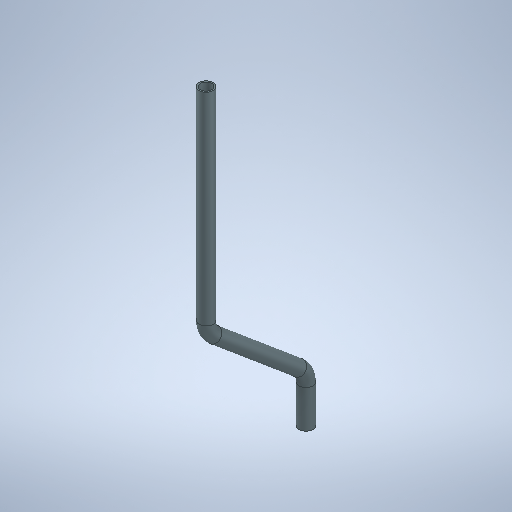
# Autodesk Inventor part: 158 diameter 76
Saved by Autodesk Inventor 2025.1 (Build 291241000, 241)
## iProperties
Created: 2024-08-03
Part Number: 158 diameter 76
Material: Iron, Gray
Document SubType Name: Modeling
Designer: ffogue
Density: 7.15 g/cm^3
Appearance: Lead
Author: ffogue
Autodesk Inventor part; units mm, degrees
ref_plane "YZ Plane" through (0, 0, 0) normal (1, 0, 0) x (0, 1, 0)
ref_plane "XZ Plane" through (0, 0, 0) normal (0, 1, 0) x (-1, 0, 0)
ref_plane "XY Plane" through (0, 0, 0) normal (0, 0, 1) x (1, 0, 0)
sketch "Sketch1" plane through (0, 0, 0) normal (0, 0, 1) x (1, 0, 0)
  circle A0 centre (0, 0) radius 2.5
  dimension "d0" = 5
  constraints: 1 centre point, 1 coincident
  measures "d0" diameter of A0
sketch "Sketch2" plane through (0, 0, 0) normal (1, 0, 0) x (0, 1, 0)
  line L0 (0, 0) -> (0, -72.5029)
  line L1 (2.6789, -78.248) -> (33.0711, -103.752)
  line L2 (35.75, -109.4971) -> (35.75, -123)
  arc A0 (0, -72.5029) -> (2.6789, -78.248) centre (7.5, -72.5029) ccw
  arc A1 (35.75, -109.4971) -> (33.0711, -103.752) centre (28.25, -109.4971) ccw
  point P0 (0, -76)
  point P1 (35.75, -106)
  dimension "d1" = 76
  dimension "d2" = 35.75
  dimension "d3" = 17
  dimension "d4" = 30
  dimension "d5" = 7.5
  constraints: 6 end point, 4 point on circle, 4 point on line, 4 tangent, 2 centre point, 1 equal radius, 1 parallel, 1 vertical
  measures "d1" distance of L0.start point (0, -76)
  measures "d2" distance between parallel lines of L0 L2
  measures "d3" distance of point (35.75, -106) L2.end
  measures "d4" vertical distance of point (35.75, -106) point (0, -76)
  measures "d5" radius of A0
sweep "Sweep1" add profiles "Sketch1" path "Sketch2"
shell "Shell1" thickness 0.5 removed faces 2 at (-0.852, 0.5526, 0) at (0.4229, 36.3026, -123)
body "Solid1"
